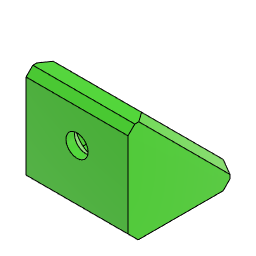
Simple Angle Bracket v5 (Autodesk Fusion 360 design; units mm, degrees)
Autodesk Fusion 360 part; units mm, degrees
sketch "Sketch1" plane through (0, 0, 0) normal (1, 0, 0) x (0, 1, 0)
  line L0 (0, 0) -> (0, 30)
  line L1 (0, 30) -> (6, 30)
  line L2 (0, 0) -> (30, 0)
  line L3 (30, 0) -> (30, 6)
  line L4 (30, 6) -> (6, 30)
  dimension "d1" = 30
  dimension "d2" = 6
  dimension "d3" = 90
  dimension "d4" = 30
  dimension "d5" = 6
  constraint coincident L0.start L2.start
  constraint vertical L0
  constraint horizontal L2
  constraint perpendicular L2 L3
  measures "d1" distance of L0.start L0.end
  measures "d2" distance of L0.end L1.end
  measures "d3" angle of L0 L1
  measures "d4" distance of L0.start L2.end
  measures "d5" distance of L2.end L3.end
extrude "Extrude1" add sketch "Sketch1" along normal blind 30
shell "Shell1" thickness 6 removed faces 3 at (10, 22, 14) at (10, 30, 2) at (10, 2, 30)
sketch "Sketch2" plane through (0, 0, 0) normal (0, 0, -1) x (1, 0, 0)
  line L0 (0, 0) -> (0, -30)
  line L1 (30, 0) -> (0, 0)
  line L2 (6, -30) -> (6, -6)
  line L3 (6, -6) -> (24, -6)
  line L4 (24, -6) -> (24, -30)
  line L5 (15, -6) -> (15, -30) construction
  circle A0 centre (15, -18) radius 3.25
  line L6 (24, -30) -> (6, -30)
  dimension "d24" = 6.5
  constraint midpoint L3 L5.start
  constraint midpoint L5 A0.centre
  constraint midpoint L5.end L6
  measures "d24" diameter of A0
extrude "Extrude3" cut sketch "Sketch2" against normal through all contours A0
ref_plane "WorkPlane1" through (15, 0, 0) normal (0, -0.707107, 0.707107) x (-1, 0, 0)
chamfer "Chamfer3" distance 3.5 angle 45 1 edges at (11.9699, 19.1753, 6)
mirror "Mirror2" about plane through (15, 0, 0) normal (0, -0.707107, 0.707107) of "Extrude3", "Chamfer3"
chamfer "Chamfer4" distance 2 angle 45 5 edges at (15, 6, 6) (24, 18, 6) (24, 6, 18) (6, 6, 18) (6, 18, 6)
chamfer "Chamfer5" distance 3 angle 45 1 edges at (15, 0, 0)
chamfer "Chamfer6" distance 2 angle 45 4 edges at (15, 0, 30) (0, 18, 18) (30, 18, 18) (15, 30, 0)
equation "d5 = d2"
